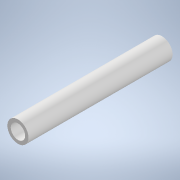
# Autodesk Inventor part: handelbar screw on extension
Saved by Autodesk Inventor 2022.2 (Build 262287000, 287)
## iProperties
Created: 2022-04-23
Part Number: handelbar screw on extension
Material: Aluminum 6061
Document SubType Name: Modeling
Designer: foriw
Density: 2.7 g/cm^3
Appearance: Black
Author: foriw
Autodesk Inventor part; units mm, degrees
ref_plane "YZ Plane" through (0, 0, 0) normal (1, 0, 0) x (0, 1, 0)
ref_plane "XZ Plane" through (0, 0, 0) normal (0, 1, 0) x (-1, 0, 0)
ref_plane "XY Plane" through (0, 0, 0) normal (0, 0, 1) x (1, 0, 0)
sketch "Sketch1" plane through (0, 0, 0) normal (0, 0, 1) x (1, 0, 0)
  circle A0 centre (0, 0) radius 7.5
  circle A1 centre (0, 0) radius 11
  dimension "d0" = 15
  dimension "d1" = 22
  constraints: 2 centre point, 2 coincident
  measures "d0" diameter of A0
  measures "d1" diameter of A1
extrude "Extrusion1" add sketch "Sketch1" along normal blind 136
extrude "Extrusion2" add sketch "Sketch1" against normal blind 14
thread "Thread1" size "M15x1.5" class "6H" standard "ANSI Metric M Profile" length 14
body "Solid1"
